Autodesk Fusion 360 part; units mm, degrees
note: some values were not read from the file. Set by a fixed rule: which sketch regions a step uses.
(part 5 of 6)
  line L3690 (386, -69.8094) -> (388, -68.6547)
  line L3691 (362, -93.3453) -> (362, -95.6547)
  line L3692 (391.5, -65.1906) -> (389.5, -66.3453)
  line L3693 (385.25, -90.8916) -> (385.25, -88.5822)
  line L3694 (396.25, -61.5822) -> (394.25, -60.4275)
  line L3695 (391.5, -65.1906) -> (389.5, -66.3453)
  line L3696 (399.75, -65.0463) -> (401.75, -63.8916)
  line L3697 (388.75, -101.0463) -> (390.75, -99.8916)
  line L3698 (388.75, -69.4275) -> (386.75, -70.5822)
  line L3699 (397, -60.8094) -> (399, -59.6547)
  line L3700 (374.25, -61.5822) -> (372.25, -60.4275)
  line L3701 (395, -59.6547) -> (397, -60.8094)
  line L3702 (402.5, -65.1906) -> (400.5, -66.3453)
  line L3703 (404.1665, -57.1527) -> (402.5, -56.1906)
  line L3704 (389.5, -93.3453) -> (389.5, -95.6547)
  line L3705 (386.75, -90.8916) -> (388.75, -92.0463)
  line L3706 (401.75, -63.8916) -> (401.75, -61.5822)
  line L3707 (366, -102.3453) -> (364, -101.1906)
  line L3708 (397.75, -61.5822) -> (397.75, -63.8916)
  line L3709 (373, -59.6547) -> (375, -60.8094)
  line L3710 (388.75, -65.0463) -> (390.75, -63.8916)
  line L3711 (379.75, -90.8916) -> (379.75, -88.5822)
  line L3712 (399.75, -60.4275) -> (397.75, -61.5822)
  line L3713 (386.75, -97.5822) -> (386.75, -99.8916)
  line L3714 (379.75, -54.8916) -> (379.75, -52.5822)
  line L3715 (373, -68.6547) -> (375, -69.8094)
  line L3716 (362, -93.3453) -> (362, -95.6547)
  line L3717 (374.25, -70.5822) -> (372.25, -69.4275)
  line L3718 (374.25, -61.5822) -> (372.25, -60.4275)
  line L3719 (397, -65.1906) -> (395, -66.3453)
  line L3720 (372.25, -65.0463) -> (374.25, -63.8916)
  line L3721 (359.25, -70.5822) -> (359.25, -72.8916)
  line L3722 (386.75, -90.8916) -> (388.75, -92.0463)
  line L3723 (379.75, -90.8916) -> (379.75, -88.5822)
  line L3724 (385.25, -54.8916) -> (385.25, -52.5822)
  line L3725 (401.75, -63.8916) -> (401.75, -61.5822)
  line L3726 (388.75, -65.0463) -> (390.75, -63.8916)
  line L3727 (386.75, -52.5822) -> (386.75, -54.8916)
  line L3728 (375.75, -52.5822) -> (375.75, -54.8916)
  line L3729 (375, -65.1906) -> (373, -66.3453)
  line L3730 (367.5, -93.3453) -> (367.5, -95.6547)
  line L3731 (372.25, -69.4275) -> (370.25, -70.5822)
  line L3732 (375.75, -88.5822) -> (375.75, -90.8916)
  line L3733 (358.5, -87.8094) -> (360.5, -86.6547)
  line L3734 (368.75, -81.8916) -> (368.75, -79.5822)
  line L3735 (364, -96.8094) -> (366, -95.6547)
  line L3736 (373, -66.3453) -> (373, -68.6547)
  line L3737 (388, -66.3453) -> (386, -65.1906)
  line L3738 (377.75, -101.0463) -> (379.75, -99.8916)
  line L3739 (392.25, -70.5822) -> (392.25, -72.8916)
  line L3740 (355.75, -87.4275) -> (353.75, -88.5822)
  line L3741 (379.75, -99.8916) -> (379.75, -97.5822)
  line L3742 (357.75, -72.8916) -> (357.75, -70.5822)
  line L3743 (394.25, -56.0463) -> (396.25, -54.8916)
  line L3744 (362, -84.3453) -> (362, -86.6547)
  line L3745 (402.5, -60.8094) -> (404.5, -59.6547)
  line L3746 (386.75, -70.5822) -> (386.75, -72.8916)
  line L3747 (386, -65.1906) -> (384, -66.3453)
  line L3748 (374.25, -72.8916) -> (374.25, -70.5822)
  line L3749 (366.75, -92.0463) -> (368.75, -90.8916)
  line L3750 (364, -92.1906) -> (362, -93.3453)
  line L3751 (356.5, -86.6547) -> (358.5, -87.8094)
  line L3752 (386.75, -88.5822) -> (386.75, -90.8916)
  line L3753 (370.25, -70.5822) -> (370.25, -72.8916)
  line L3754 (374.25, -72.8916) -> (374.25, -70.5822)
  line L3755 (386.75, -52.5822) -> (386.75, -54.8916)
  line L3756 (390.75, -90.8916) -> (390.75, -88.5822)
  line L3757 (370.25, -70.5822) -> (370.25, -72.8916)
  line L3758 (378.5, -93.3453) -> (378.5, -95.6547)
  line L3759 (366.75, -101.0463) -> (368.75, -99.8916)
  line L3760 (358.5, -83.1906) -> (356.5, -84.3453)
  line L3761 (360.5, -84.3453) -> (358.5, -83.1906)
  line L3762 (397.75, -54.8916) -> (399.75, -56.0463)
  line L3763 (392.25, -88.5822) -> (392.25, -90.8916)
  line L3764 (360.5, -84.3453) -> (358.5, -83.1906)
  line L3765 (394.25, -56.0463) -> (396.25, -54.8916)
  line L3766 (388, -66.3453) -> (386, -65.1906)
  line L3767 (360.5, -86.6547) -> (360.5, -84.3453)
  line L3768 (389.5, -66.3453) -> (389.5, -68.6547)
  line L3769 (368.75, -97.5822) -> (366.75, -96.4275)
  line L3770 (385.25, -54.8916) -> (385.25, -52.5822)
  line L3771 (404.5, -66.3453) -> (402.5, -65.1906)
  line L3772 (379.75, -54.8916) -> (379.75, -52.5822)
  line L3773 (377.75, -92.0463) -> (379.75, -90.8916)
  line L3774 (399.75, -56.0463) -> (401.75, -54.8916)
  line L3775 (355, -86.6547) -> (355, -84.3453)
  line L3776 (401.75, -54.8916) -> (401.75, -53.9293)
  line L3777 (363.25, -81.8916) -> (363.25, -79.5822)
  line L3778 (390.75, -70.5822) -> (388.75, -69.4275)
  line L3779 (401.75, -54.8916) -> (401.75, -53.9293)
  line L3780 (385.25, -72.8916) -> (385.25, -70.5822)
  line L3781 (373, -66.3453) -> (373, -68.6547)
  line L3782 (390.75, -90.8916) -> (390.75, -88.5822)
  line L3783 (372.25, -60.4275) -> (370.25, -61.5822)
  line L3784 (370.25, -61.5822) -> (370.25, -63.8916)
  line L3785 (384, -66.3453) -> (384, -68.6547)
  line L3786 (366.75, -92.0463) -> (368.75, -90.8916)
  line L3787 (364, -92.1906) -> (362, -93.3453)
  line L3788 (360.5, -86.6547) -> (360.5, -84.3453)
  line L3789 (364, -101.1906) -> (362, -102.3453)
  line L3790 (367.5, -93.3453) -> (367.5, -95.6547)
  line L3791 (366.75, -101.0463) -> (368.75, -99.8916)
  line L3792 (370.25, -79.5822) -> (370.25, -81.8916)
  line L3793 (363.25, -99.8916) -> (363.25, -97.5822)
  line L3794 (364.75, -79.5822) -> (364.75, -81.8916)
  line L3795 (386.75, -88.5822) -> (386.75, -90.8916)
  line L3796 (379.75, -97.5822) -> (377.75, -96.4275)
  line L3797 (364.75, -97.5822) -> (364.75, -99.8916)
  line L3798 (392.25, -70.5822) -> (392.25, -72.8916)
  line L3799 (375.75, -88.5822) -> (375.75, -90.8916)
  line L3800 (374.25, -81.8916) -> (374.25, -79.5822)
  line L3801 (390.75, -72.8916) -> (390.75, -70.5822)
  line L3802 (366, -93.3453) -> (364, -92.1906)
  line L3803 (364.75, -90.8916) -> (366.75, -92.0463)
  line L3804 (381.25, -52.5822) -> (381.25, -54.8916)
  line L3805 (375.75, -97.5822) -> (375.75, -99.8916)
  line L3806 (366, -95.6547) -> (366, -93.3453)
  line L3807 (375.75, -97.5822) -> (375.75, -99.8916)
  line L3808 (386.75, -63.8916) -> (388.75, -65.0463)
  line L3809 (377, -95.6547) -> (377, -93.3453)
  line L3810 (359.25, -81.8916) -> (361.25, -83.0463)
  line L3811 (375.75, -90.8916) -> (377.75, -92.0463)
  line L3812 (399, -59.6547) -> (399, -57.3453)
  line L3813 (368.75, -99.8916) -> (368.75, -97.5822)
  line L3814 (377.75, -96.4275) -> (375.75, -97.5822)
  line L3815 (397, -56.1906) -> (395, -57.3453)
  line L3816 (382.5, -93.3453) -> (380.5, -92.1906)
  line L3817 (352.25, -72.8916) -> (352.25, -70.5822)
  line L3818 (359.25, -81.8916) -> (361.25, -83.0463)
  line L3819 (361.25, -87.4275) -> (359.25, -88.5822)
  line L3820 (400.5, -59.6547) -> (402.5, -60.8094)
  line L3821 (399, -57.3453) -> (397, -56.1906)
  line L3822 (397.75, -54.8916) -> (399.75, -56.0463)
  line L3823 (348.25, -70.5822) -> (348.25, -72.8916)
  line L3824 (362, -84.3453) -> (362, -86.6547)
  line L3825 (397, -56.1906) -> (395, -57.3453)
  line L3826 (399, -57.3453) -> (397, -56.1906)
  line L3827 (378.5, -95.6547) -> (380.5, -96.8094)
  line L3828 (378.5, -95.6547) -> (380.5, -96.8094)
  line L3829 (366.75, -96.4275) -> (364.75, -97.5822)
  line L3830 (388, -68.6547) -> (388, -66.3453)
  line L3831 (389.5, -68.6547) -> (391.5, -69.8094)
  line L3832 (364.75, -97.5822) -> (364.75, -99.8916)
  line L3833 (377.75, -92.0463) -> (379.75, -90.8916)
  line L3834 (381.25, -90.8916) -> (383.25, -92.0463)
  line L3835 (386.75, -63.8916) -> (388.75, -65.0463)
  line L3836 (355, -86.6547) -> (355, -84.3453)
  line L3837 (381.25, -88.5822) -> (381.25, -90.8916)
  line L3838 (366.75, -96.4275) -> (364.75, -97.5822)
  line L3839 (399.75, -56.0463) -> (401.75, -54.8916)
  line L3840 (363.25, -81.8916) -> (363.25, -79.5822)
  line L3841 (390.75, -72.8916) -> (390.75, -70.5822)
  line L3842 (377, -95.6547) -> (377, -93.3453)
  line L3843 (369.5, -60.8094) -> (371.5, -59.6547)
  line L3844 (361.25, -87.4275) -> (359.25, -88.5822)
  line L3845 (388, -68.6547) -> (388, -66.3453)
  line L3846 (362, -95.6547) -> (364, -96.8094)
  line L3847 (368.75, -99.8916) -> (368.75, -97.5822)
  line L3848 (385.25, -72.8916) -> (385.25, -70.5822)
  line L3849 (364.75, -79.5822) -> (364.75, -81.8916)
  line L3850 (389.5, -68.6547) -> (391.5, -69.8094)
  line L3851 (371.5, -66.3453) -> (369.5, -65.1906)
  line L3852 (356.5, -86.6547) -> (358.5, -87.8094)
  line L3853 (366, -102.3453) -> (364, -101.1906)
  line L3854 (364.75, -90.8916) -> (366.75, -92.0463)
  line L3855 (364, -96.8094) -> (366, -95.6547)
  line L3856 (399, -59.6547) -> (399, -57.3453)
  line L3857 (353.75, -81.8916) -> (355.75, -83.0463)
  line L3858 (358.5, -83.1906) -> (356.5, -84.3453)
  line L3859 (366, -93.3453) -> (364, -92.1906)
  line L3860 (393.5, -59.6547) -> (393.5, -57.3453)
  line L3861 (358.5, -87.8094) -> (360.5, -86.6547)
  line L3862 (384, -68.6547) -> (386, -69.8094)
  line L3863 (364.75, -99.8916) -> (366.75, -101.0463)
  line L3864 (371.5, -57.3453) -> (369.5, -56.1906)
  line L3865 (381.25, -52.5822) -> (381.25, -54.8916)
  line L3866 (357.75, -88.5822) -> (355.75, -87.4275)
  line L3867 (373, -41.6547) -> (375, -42.8094)
  line L3868 (381.25, -97.5822) -> (381.25, -99.8916)
  line L3869 (364, -101.1906) -> (362, -102.3453)
  line L3870 (372.25, -42.4275) -> (370.25, -43.5822)
  line L3871 (355.75, -83.0463) -> (357.75, -81.8916)
  line L3872 (372.25, -51.4275) -> (370.25, -52.5822)
  line L3873 (380.5, -92.1906) -> (378.5, -93.3453)
  line L3874 (393.5, -59.6547) -> (393.5, -57.3453)
  line L3875 (369.5, -51.8094) -> (371.5, -50.6547)
  line L3876 (392.25, -52.5822) -> (392.25, -54.8916)
  line L3877 (372.25, -42.4275) -> (370.25, -43.5822)
  line L3878 (357.75, -72.8916) -> (357.75, -70.5822)
  line L3879 (386.75, -70.5822) -> (386.75, -72.8916)
  line L3880 (388.75, -69.4275) -> (386.75, -70.5822)
  line L3881 (366, -95.6547) -> (366, -93.3453)
  line L3882 (355.75, -83.0463) -> (357.75, -81.8916)
  line L3883 (375.75, -90.8916) -> (377.75, -92.0463)
  line L3884 (368.75, -97.5822) -> (366.75, -96.4275)
  line L3885 (386, -65.1906) -> (384, -66.3453)
  line L3886 (384, -66.3453) -> (384, -68.6547)
  line L3887 (383.25, -78.4275) -> (381.25, -79.5822)
  line L3888 (390.75, -70.5822) -> (388.75, -69.4275)
  line L3889 (375, -56.1906) -> (373, -57.3453)
  line L3890 (381.25, -99.8916) -> (383.25, -101.0463)
  line L3891 (357.75, -88.5822) -> (355.75, -87.4275)
  line L3892 (402.5, -56.1906) -> (400.5, -57.3453)
  line L3893 (374.25, -45.8916) -> (374.25, -43.5822)
  line L3894 (371.5, -57.3453) -> (369.5, -56.1906)
  line L3895 (356.5, -84.3453) -> (356.5, -86.6547)
  line L3896 (380.5, -96.8094) -> (382.5, -95.6547)
  line L3897 (379.75, -99.8916) -> (379.75, -97.5822)
  line L3898 (370.25, -52.5822) -> (370.25, -54.8916)
  line L3899 (404.5, -66.3453) -> (402.5, -65.1906)
  line L3900 (400.5, -57.3453) -> (400.5, -59.6547)
  line L3901 (402.5, -56.1906) -> (400.5, -57.3453)
  line L3902 (371.5, -50.6547) -> (371.5, -48.3453)
  line L3903 (356.5, -84.3453) -> (356.5, -86.6547)
  line L3904 (382.5, -95.6547) -> (382.5, -93.3453)
  line L3905 (362, -95.6547) -> (364, -96.8094)
  line L3906 (381.25, -97.5822) -> (381.25, -99.8916)
  line L3907 (386, -69.8094) -> (388, -68.6547)
  line L3908 (395, -57.3453) -> (395, -59.6547)
  line L3909 (382.5, -93.3453) -> (380.5, -92.1906)
  line L3910 (355.75, -87.4275) -> (353.75, -88.5822)
  line L3911 (377.75, -101.0463) -> (379.75, -99.8916)
  line L3912 (353.75, -70.5822) -> (353.75, -72.8916)
  line L3913 (364.75, -99.8916) -> (366.75, -101.0463)
  line L3914 (389.5, -66.3453) -> (389.5, -68.6547)
  line L3915 (400.5, -59.6547) -> (402.5, -60.8094)
  line L3916 (400.5, -57.3453) -> (400.5, -59.6547)
  line L3917 (374.25, -52.5822) -> (372.25, -51.4275)
  line L3918 (381.25, -81.8916) -> (383.25, -83.0463)
  line L3919 (370.25, -43.5822) -> (370.25, -45.8916)
  line L3920 (369.5, -60.8094) -> (371.5, -59.6547)
  line L3921 (395, -57.3453) -> (395, -59.6547)
  line L3922 (375.75, -99.8916) -> (377.75, -101.0463)
  line L3923 (383.25, -87.4275) -> (381.25, -88.5822)
  line L3924 (352.25, -72.8916) -> (352.25, -70.5822)
  line L3925 (346.75, -72.8916) -> (346.75, -70.5822)
  line L3926 (375.75, -52.5822) -> (375.75, -54.8916)
  line L3927 (346.75, -72.8916) -> (346.75, -70.5822)
  line L3928 (370.25, -43.5822) -> (370.25, -45.8916)
  line L3929 (356.5, -77.6547) -> (358.5, -78.8094)
  line L3930 (378.5, -93.3453) -> (378.5, -95.6547)
  line L3931 (385.25, -88.5822) -> (383.25, -87.4275)
  line L3932 (370.25, -45.8916) -> (372.25, -47.0463)
  line L3933 (372.25, -47.0463) -> (374.25, -45.8916)
  line L3934 (369.5, -42.8094) -> (371.4564, -41.6798)
  line L3935 (388.75, -87.4275) -> (386.75, -88.5822)
  line L3936 (379.75, -97.5822) -> (377.75, -96.4275)
  line L3937 (390.75, -88.5822) -> (388.75, -87.4275)
  line L3938 (375, -56.1906) -> (373, -57.3453)
  line L3939 (353, -78.8094) -> (355, -77.6547)
  line L3940 (348.25, -70.5822) -> (348.25, -72.8916)
  line L3941 (386, -83.1906) -> (384, -84.3453)
  line L3942 (372.25, -56.0463) -> (374.25, -54.8916)
  line L3943 (355, -75.3453) -> (353, -74.1906)
  line L3944 (371.5, -75.3453) -> (369.5, -74.1906)
  line L3945 (384, -84.3453) -> (384, -86.6547)
  line L3946 (369.5, -42.8094) -> (371.4564, -41.6798)
  line L3947 (385.25, -97.5822) -> (383.25, -96.4275)
  line L3948 (361.25, -78.4275) -> (359.25, -79.5822)
  line L3949 (381.25, -90.8916) -> (383.25, -92.0463)
  line L3950 (375, -47.1906) -> (373, -48.3453)
  line L3951 (372.25, -56.0463) -> (374.25, -54.8916)
  line L3952 (374.25, -54.8916) -> (374.25, -52.5822)
  line L3953 (355.75, -78.4275) -> (353.75, -79.5822)
  line L3954 (383.25, -92.0463) -> (385.25, -90.8916)
  line L3955 (385.25, -79.5822) -> (383.25, -78.4275)
  line L3956 (381.25, -99.8916) -> (383.25, -101.0463)
  line L3957 (380.5, -92.1906) -> (378.5, -93.3453)
  line L3958 (382.5, -68.6547) -> (382.5, -66.3453)
  line L3959 (352.25, -54.8916) -> (352.25, -52.5822)
  line L3960 (357.75, -79.5822) -> (355.75, -78.4275)
  line L3961 (389.5, -84.3453) -> (389.5, -86.6547)
  line L3962 (370.25, -45.8916) -> (372.25, -47.0463)
  line L3963 (373, -41.5572) -> (373, -41.6547)
  line L3964 (385.25, -79.5822) -> (383.25, -78.4275)
  line L3965 (375.75, -99.8916) -> (377.75, -101.0463)
  line L3966 (383.25, -83.0463) -> (385.25, -81.8916)
  line L3967 (386.75, -81.8916) -> (388.75, -83.0463)
  line L3968 (383.25, -87.4275) -> (381.25, -88.5822)
  line L3969 (388, -86.6547) -> (388, -84.3453)
  line L3970 (382.5, -95.6547) -> (382.5, -93.3453)
  line L3971 (375.75, -70.5822) -> (375.75, -72.8916)
  line L3972 (383.25, -96.4275) -> (381.25, -97.5822)
  line L3973 (383.25, -96.4275) -> (381.25, -97.5822)
  line L3974 (377.75, -65.0463) -> (379.75, -63.8916)
  line L3975 (381.25, -70.5822) -> (381.25, -72.8916)
  line L3976 (383.25, -101.0463) -> (385.25, -99.8916)
  line L3977 (377.75, -96.4275) -> (375.75, -97.5822)
  line L3978 (381.25, -81.8916) -> (383.25, -83.0463)
  line L3979 (355, -77.6547) -> (355, -75.3453)
  line L3980 (383.25, -83.0463) -> (385.25, -81.8916)
  line L3981 (359.25, -70.5822) -> (359.25, -72.8916)
  line L3982 (388, -86.6547) -> (388, -84.3453)
  line L3983 (353, -78.8094) -> (355, -77.6547)
  line L3984 (360.5, -75.3453) -> (358.5, -74.1906)
  line L3985 (390.75, -88.5822) -> (388.75, -87.4275)
  arc A135 (371.4564, -41.6798) -> (368.3398, -42.1395) centre (375, -76.5) ccw
  line L3986 (388, -84.3453) -> (386, -83.1906)
  line L3987 (369.5, -69.8094) -> (371.5, -68.6547)
  line L3988 (373, -48.3453) -> (373, -50.6547)
  line L3989 (380.5, -96.8094) -> (382.5, -95.6547)
  line L3990 (382.5, -68.6547) -> (382.5, -66.3453)
  line L3991 (389.5, -84.3453) -> (389.5, -86.6547)
  line L3992 (373, -50.6547) -> (375, -51.8094)
  line L3993 (383.25, -101.0463) -> (385.25, -99.8916)
  line L3994 (358.5, -74.1906) -> (356.5, -75.3453)
  line L3995 (360.5, -77.6547) -> (360.5, -75.3453)
  line L3996 (358.5, -78.8094) -> (360.5, -77.6547)
  line L3997 (370.25, -54.8916) -> (372.25, -56.0463)
  line L3998 (375.75, -70.5822) -> (375.75, -72.8916)
  line L3999 (371.5, -50.6547) -> (371.5, -48.3453)
  line L4000 (389.5, -86.6547) -> (391.5, -87.8094)
  line L4001 (375.75, -63.8916) -> (377.75, -65.0463)
  line L4002 (388.75, -83.0463) -> (390.75, -81.8916)
  line L4003 (386, -87.8094) -> (388, -86.6547)
  line L4004 (379.75, -72.8916) -> (379.75, -70.5822)
  line L4005 (378.5, -66.3453) -> (378.5, -68.6547)
  line L4006 (374.25, -45.8916) -> (374.25, -43.5822)
  line L4007 (386.75, -61.5822) -> (386.75, -63.8916)
  line L4008 (389.5, -86.6547) -> (391.5, -87.8094)
  line L4009 (370.25, -54.8916) -> (372.25, -56.0463)
  line L4010 (362, -75.3453) -> (362, -77.6547)
  line L4011 (384, -84.3453) -> (384, -86.6547)
  line L4012 (360.5, -75.3453) -> (358.5, -74.1906)
  line L4013 (379.75, -45.8916) -> (379.75, -43.5822)
  line L4014 (369.5, -78.8094) -> (371.5, -77.6547)
  line L4015 (358.5, -74.1906) -> (356.5, -75.3453)
  line L4016 (377, -68.6547) -> (377, -66.3453)
  line L4017 (388.75, -87.4275) -> (386.75, -88.5822)
  line L4018 (360.5, -68.6547) -> (360.5, -66.3453)
  line L4019 (391.5, -83.1906) -> (389.5, -84.3453)
  line L4020 (383.25, -78.4275) -> (381.25, -79.5822)
  line L4021 (372.25, -47.0463) -> (374.25, -45.8916)
  line L4022 (371.5, -66.3453) -> (369.5, -65.1906)
  line L4023 (355, -84.3453) -> (353, -83.1906)
  line L4024 (359.25, -52.5822) -> (359.25, -54.8916)
  line L4025 (391.5, -83.1906) -> (389.5, -84.3453)
  line L4026 (374.25, -43.5822) -> (372.25, -42.4275)
  line L4027 (377.75, -69.4275) -> (375.75, -70.5822)
  line L4028 (386, -87.8094) -> (388, -86.6547)
  line L4029 (348.25, -53.9293) -> (348.25, -54.8916)
  line L4030 (374.25, -54.8916) -> (374.25, -52.5822)
  line L4031 (381.25, -70.5822) -> (381.25, -72.8916)
  line L4032 (385.25, -88.5822) -> (383.25, -87.4275)
  line L4033 (373, -41.5572) -> (373, -41.6547)
  line L4034 (380.5, -69.8094) -> (382.5, -68.6547)
  line L4035 (355.75, -65.0463) -> (357.75, -63.8916)
  line L4036 (382.5, -66.3453) -> (380.5, -65.1906)
  line L4037 (355.75, -78.4275) -> (353.75, -79.5822)
  line L4038 (369.5, -51.8094) -> (371.5, -50.6547)
  line L4039 (371.5, -75.3453) -> (369.5, -74.1906)
  line L4040 (369.5, -78.8094) -> (371.5, -77.6547)
  line L4041 (353.75, -72.8916) -> (355.75, -74.0463)
  line L4042 (373, -50.6547) -> (375, -51.8094)
  line L4043 (379.75, -72.8916) -> (379.75, -70.5822)
  line L4044 (357.75, -54.8916) -> (357.75, -52.5822)
  line L4045 (358.5, -78.8094) -> (360.5, -77.6547)
  line L4046 (383.25, -92.0463) -> (385.25, -90.8916)
  line L4047 (390.75, -81.8916) -> (390.75, -79.5822)
  line L4048 (385.25, -97.5822) -> (383.25, -96.4275)
  line L4049 (373, -48.3453) -> (373, -50.6547)
  line L4050 (356.5, -66.3453) -> (356.5, -68.6547)
  line L4051 (353, -87.8094) -> (355, -86.6547)
  line L4052 (355, -77.6547) -> (355, -75.3453)
  line L4053 (384, -86.6547) -> (386, -87.8094)
  line L4054 (377, -68.6547) -> (377, -66.3453)
  line L4055 (382.5, -84.3453) -> (380.5, -83.1906)
  line L4056 (388, -84.3453) -> (386, -83.1906)
  line L4057 (373, -57.3453) -> (373, -59.6547)
  line L4058 (388, -48.3453) -> (386, -47.1906)
  line L4059 (360.5, -77.6547) -> (360.5, -75.3453)
  line L4060 (372.25, -51.4275) -> (370.25, -52.5822)
  line L4061 (379.75, -63.8916) -> (379.75, -61.5822)
  line L4062 (359.25, -72.8916) -> (361.25, -74.0463)
  line L4063 (357.75, -70.5822) -> (355.75, -69.4275)
  line L4064 (392.25, -79.5822) -> (392.25, -81.8916)
  line L4065 (375, -47.1906) -> (373, -48.3453)
  line L4066 (356.5, -68.6547) -> (358.5, -69.8094)
  line L4067 (362, -66.3453) -> (362, -68.6547)
  line L4068 (373, -41.6547) -> (375, -42.8094)
  line L4069 (362, -66.3453) -> (362, -68.6547)
  line L4070 (355.75, -74.0463) -> (357.75, -72.8916)
  line L4071 (375.75, -63.8916) -> (377.75, -65.0463)
  line L4072 (378.5, -86.6547) -> (380.5, -87.8094)
  line L4073 (356.5, -68.6547) -> (358.5, -69.8094)
  line L4074 (382.5, -84.3453) -> (380.5, -83.1906)
  line L4075 (386, -83.1906) -> (384, -84.3453)
  line L4076 (359.25, -63.8916) -> (361.25, -65.0463)
  line L4077 (392.25, -79.5822) -> (392.25, -81.8916)
  line L4078 (384, -86.6547) -> (386, -87.8094)
  line L4079 (386.75, -45.8916) -> (388.75, -47.0463)
  line L4080 (378.5, -68.6547) -> (380.5, -69.8094)
  line L4081 (359.25, -63.8916) -> (361.25, -65.0463)
  line L4082 (385.25, -81.8916) -> (385.25, -79.5822)
  line L4083 (386, -47.1906) -> (384, -48.3453)
  line L4084 (377, -86.6547) -> (377, -84.3453)
  line L4085 (371.5, -59.6547) -> (371.5, -57.3453)
  line L4086 (380.5, -69.8094) -> (382.5, -68.6547)
  line L4087 (379.75, -70.5822) -> (377.75, -69.4275)
  line L4088 (374.25, -43.5822) -> (372.25, -42.4275)
  line L4089 (381.25, -43.5822) -> (381.25, -45.8916)
  line L4090 (357.75, -79.5822) -> (355.75, -78.4275)
  line L4091 (379.75, -63.8916) -> (379.75, -61.5822)
  line L4092 (359.25, -72.8916) -> (361.25, -74.0463)
  line L4093 (386.75, -81.8916) -> (388.75, -83.0463)
  line L4094 (361.25, -69.4275) -> (359.25, -70.5822)
  line L4095 (389.5, -50.6547) -> (391.5, -51.8094)
  line L4096 (380.5, -65.1906) -> (378.5, -66.3453)
  line L4097 (357.75, -70.5822) -> (355.75, -69.4275)
  line L4098 (390.75, -81.8916) -> (390.75, -79.5822)
  line L4099 (361.25, -78.4275) -> (359.25, -79.5822)
  line L4100 (375.75, -43.5822) -> (375.75, -45.8916)
  line L4101 (374.25, -52.5822) -> (372.25, -51.4275)
  line L4102 (375.75, -81.8916) -> (377.75, -83.0463)
  line L4103 (370.25, -52.5822) -> (370.25, -54.8916)
  line L4104 (382.5, -66.3453) -> (380.5, -65.1906)
  line L4105 (381.25, -43.5822) -> (381.25, -45.8916)
  line L4106 (377.75, -65.0463) -> (379.75, -63.8916)
  line L4107 (388.75, -83.0463) -> (390.75, -81.8916)
  line L4108 (356.5, -75.3453) -> (356.5, -77.6547)
  line L4109 (362, -75.3453) -> (362, -77.6547)
  line L4110 (373, -57.3453) -> (373, -59.6547)
  line L4111 (377.75, -87.4275) -> (375.75, -88.5822)
  line L4112 (379.75, -70.5822) -> (377.75, -69.4275)
  line L4113 (378.5, -68.6547) -> (380.5, -69.8094)
  line L4114 (356.5, -75.3453) -> (356.5, -77.6547)
  line L4115 (361.25, -69.4275) -> (359.25, -70.5822)
  arc A136 (371.4564, -41.6798) -> (368.3398, -42.1395) centre (375, -76.5) ccw
  line L4116 (379.75, -88.5822) -> (377.75, -87.4275)
  line L4117 (380.5, -65.1906) -> (378.5, -66.3453)
  line L4118 (355.75, -74.0463) -> (357.75, -72.8916)
  line L4119 (360.5, -66.3453) -> (358.5, -65.1906)
  line L4120 (377.75, -69.4275) -> (375.75, -70.5822)
  line L4121 (382.5, -86.6547) -> (382.5, -84.3453)
  line L4122 (353.75, -52.5822) -> (353.75, -54.8916)
  line L4123 (356.5, -77.6547) -> (358.5, -78.8094)
  line L4124 (388.75, -51.4275) -> (386.75, -52.5822)
  line L4125 (389.5, -48.3453) -> (389.5, -50.6547)
  line L4126 (371.5, -59.6547) -> (371.5, -57.3453)
  line L4127 (353.75, -63.8916) -> (355.75, -65.0463)
  arc A137 (387.3612, -109.2445) -> (390.75, -107.756) centre (375, -76.5) ccw
  arc A138 (387.3612, -109.2445) -> (390.75, -107.756) centre (375, -76.5) ccw
  line L4128 (388.75, -105.4275) -> (386.75, -106.5822)
  line L4129 (390.75, -106.5822) -> (388.75, -105.4275)
  line L4130 (384, -104.6547) -> (386, -105.8094)
  line L4131 (388, -104.6547) -> (388, -102.3453)
  line L4132 (380.5, -105.8094) -> (382.5, -104.6547)
  line L4133 (381.25, -106.5822) -> (381.25, -108.8916)
  line L4134 (386.75, -106.5822) -> (386.75, -108.8916)
  line L4135 (380.5, -105.8094) -> (382.5, -104.6547)
  line L4136 (375.75, -106.5822) -> (375.75, -108.8916)
  line L4137 (386, -105.8094) -> (388, -104.6547)
  line L4138 (379.75, -106.5822) -> (377.75, -105.4275)
  line L4139 (379.75, -108.8916) -> (379.75, -106.5822)
  line L4140 (386.75, -106.5822) -> (386.75, -108.8916)
  line L4141 (375.75, -106.5822) -> (375.75, -108.8916)
  line L4142 (381.25, -106.5822) -> (381.25, -108.8916)
  line L4143 (388.75, -105.4275) -> (386.75, -106.5822)
  line L4144 (379.75, -108.8916) -> (379.75, -106.5822)
  line L4145 (385.25, -108.8916) -> (385.25, -106.5822)
  line L4146 (375, -60.8094) -> (377, -59.6547)
  line L4147 (390.75, -106.5822) -> (388.75, -105.4275)
  line L4148 (385.25, -108.8916) -> (385.25, -106.5822)
  line L4149 (402.5, -96.8094) -> (404.1665, -95.8473)
  line L4150 (400.5, -95.6547) -> (402.5, -96.8094)
  line L4151 (404.5, -93.3453) -> (402.5, -92.1906)
  line L4152 (402.5, -87.8094) -> (404.5, -86.6547)
  line L4153 (400.5, -95.6547) -> (402.5, -96.8094)
  line L4154 (402.5, -92.1906) -> (400.5, -93.3453)
  line L4155 (404.5, -93.3453) -> (402.5, -92.1906)
  line L4156 (400.5, -86.6547) -> (402.5, -87.8094)
  line L4157 (395, -93.3453) -> (395, -95.6547)
  line L4158 (399, -95.6547) -> (399, -93.3453)
  line L4159 (395, -93.3453) -> (395, -95.6547)
  line L4160 (393.5, -95.6547) -> (393.5, -93.3453)
  line L4161 (400.5, -93.3453) -> (400.5, -95.6547)
  line L4162 (402.5, -92.1906) -> (400.5, -93.3453)
  line L4163 (393.5, -95.6547) -> (393.5, -93.3453)
  line L4164 (402.5, -87.8094) -> (404.5, -86.6547)
  line L4165 (400.5, -93.3453) -> (400.5, -95.6547)
  line L4166 (391.5, -105.8094) -> (393.5, -104.6547)
  line L4167 (389.5, -104.6547) -> (391.5, -105.8094)
  line L4168 (393.5, -104.6547) -> (393.5, -102.3453)
  line L4169 (390.75, -107.756) -> (390.75, -106.5822)
  line L4170 (393.5, -104.6547) -> (393.5, -102.3453)
  line L4171 (392.25, -106.5822) -> (392.25, -106.9539)
  line L4172 (391.5, -105.8094) -> (393.5, -104.6547)
  line L4173 (390.75, -107.756) -> (390.75, -106.5822)
  line L4174 (389.5, -104.6547) -> (391.5, -105.8094)
  line L4175 (389.5, -102.3453) -> (389.5, -104.6547)
  line L4176 (392.25, -106.5822) -> (392.25, -106.9539)
  line L4177 (399.75, -87.4275) -> (397.75, -88.5822)
  line L4178 (399.75, -92.0463) -> (401.75, -90.8916)
  line L4179 (397, -92.1906) -> (395, -93.3453)
  line L4180 (395, -86.6547) -> (397, -87.8094)
  line L4181 (394.25, -92.0463) -> (396.25, -90.8916)
  line L4182 (395, -86.6547) -> (397, -87.8094)
  line L4183 (397.75, -88.5822) -> (397.75, -90.8916)
  line L4184 (401.75, -90.8916) -> (401.75, -88.5822)
  line L4185 (396.25, -90.8916) -> (396.25, -88.5822)
  line L4186 (397, -87.8094) -> (399, -86.6547)
  line L4187 (401.75, -88.5822) -> (399.75, -87.4275)
  line L4188 (397, -87.8094) -> (399, -86.6547)
  line L4189 (397.75, -88.5822) -> (397.75, -90.8916)
  line L4190 (397.75, -90.8916) -> (399.75, -92.0463)
  line L4191 (397, -92.1906) -> (395, -93.3453)
  line L4192 (399, -95.6547) -> (399, -93.3453)
  line L4193 (399, -93.3453) -> (397, -92.1906)
  line L4194 (399.75, -87.4275) -> (397.75, -88.5822)
  line L4195 (399.75, -92.0463) -> (401.75, -90.8916)
  line L4196 (396.25, -88.5822) -> (394.25, -87.4275)
  line L4197 (394.25, -92.0463) -> (396.25, -90.8916)
  line L4198 (405.25, -87.4275) -> (403.25, -88.5822)
  line L4199 (405.25, -87.4275) -> (403.25, -88.5822)
  line L4200 (403.25, -90.8916) -> (405.25, -92.0463)
  arc A139 (377, -41.5572) -> (373, -41.5572) centre (375, -76.5) ccw
  line L4201 (403.25, -88.5822) -> (403.25, -90.8916)
  line L4202 (407.25, -88.5822) -> (405.25, -87.4275)
  arc A140 (406.7807, -91.1625) -> (407.25, -90.0992) centre (375, -76.5) ccw
  arc A141 (406.7807, -91.1625) -> (407.25, -90.0992) centre (375, -76.5) ccw
  line L4203 (405.25, -92.0463) -> (406.7807, -91.1625)
  line L4204 (408, -87.8094) -> (408.1524, -87.7214)
  line L4205 (407.25, -90.0992) -> (407.25, -88.5822)
  arc A142 (404.1665, -95.8473) -> (404.5, -95.3348) centre (375, -76.5) ccw
  line L4206 (403.25, -88.5822) -> (403.25, -90.8916)
  line L4207 (406, -86.6547) -> (408, -87.8094)
  line L4208 (403.25, -90.8916) -> (405.25, -92.0463)
  arc A143 (404.1665, -95.8473) -> (404.5, -95.3348) centre (375, -76.5) ccw
  line L4209 (405.25, -92.0463) -> (406.7807, -91.1625)
  line L4210 (407.25, -88.5822) -> (405.25, -87.4275)
  line L4211 (408, -87.8094) -> (408.1524, -87.7214)
  line L4212 (404.5, -95.3348) -> (404.5, -93.3453)
  line L4213 (406, -86.6547) -> (408, -87.8094)
  line L4214 (404.5, -95.3348) -> (404.5, -93.3453)
  line L4215 (407.25, -90.0992) -> (407.25, -88.5822)
  line L4216 (547.7721, 225.15) -> (517.5279, 225.15)
  arc A144 (553.8, 219.1221) -> (547.7721, 225.15) centre (532.65, 204) ccw
  line L4217 (553.8, 219.1221) -> (553.8, 188.8779)
  arc A145 (547.7721, 182.85) -> (553.8, 188.8779) centre (532.65, 204) ccw
  line L4218 (547.7721, 182.85) -> (517.5279, 182.85)
  arc A146 (511.5, 188.8779) -> (517.5279, 182.85) centre (532.65, 204) ccw
  line L4219 (511.5, 188.8779) -> (511.5, 219.1221)
  circle A147 centre (517.15, 188.5) radius 1.5
  circle A148 centre (548.15, 188.5) radius 1.5
  circle A149 centre (517.15, 219.5) radius 1.5
  circle A150 centre (548.15, 219.5) radius 1.5
  arc A151 (517.5279, 225.15) -> (511.5, 219.1221) centre (532.65, 204) ccw
  circle A152 centre (405.0052, 247.5049) radius 2
  circle A153 centre (345.0052, 247.5049) radius 2
  circle A154 centre (345.0052, 187.5049) radius 2
  circle A155 centre (405.0052, 187.5049) radius 2
  circle A156 centre (345.0026, -46.496) radius 2
  circle A157 centre (405.0026, -46.496) radius 2
  circle A158 centre (345.0026, -106.496) radius 2
  circle A159 centre (405.0026, -106.496) radius 2
  line L4220 (641.1, -21.5) -> (730.1, -21.5)
  line L4221 (730.1, -21.5) -> (730.1, -63.5)
  line L4222 (730.1, -63.5) -> (641.1, -63.5)
  line L4223 (641.1, -63.5) -> (641.1, -21.5)
  line L4224 (635.6, -119.5) -> (645.6, -119.5)
  line L4225 (645.6, -119.5) -> (645.6, -94)
  line L4226 (645.6, -94) -> (635.6, -94)
  line L4227 (635.6, -94) -> (635.6, -119.5)
  line L4228 (723.6, -94) -> (733.6, -94)
  line L4229 (733.6, -94) -> (733.6, -119.5)
  line L4230 (733.6, -119.5) -> (723.6, -119.5)
  line L4231 (723.6, -119.5) -> (723.6, -94)
  circle A160 centre (684.6183, -98.5274) radius 17.5
  line L4232 (620, -10) -> (749.2, -10)
  line L4233 (699.45, -122) -> (699.45, -125)
  line L4234 (721.95, -122) -> (744.4305, -122)
  line L4235 (749.2, -122) -> (749.2, -10)
  line L4236 (676.95, -122) -> (699.45, -122)
  line L4237 (721.95, -125) -> (721.95, -122)
  line L4238 (620, -125) -> (631.95, -125)
  line L4239 (631.95, -125) -> (631.95, -122)
  line L4240 (631.95, -122) -> (654.45, -122)
  line L4241 (744.4305, -122) -> (749.2, -122)
  line L4242 (620, -10) -> (620, -125)
  line L4243 (676.95, -125) -> (676.95, -122)
  line L4244 (654.45, -122) -> (654.45, -125)
  line L4245 (654.45, -125) -> (676.95, -125)
  line L4246 (699.45, -125) -> (721.95, -125)
  line L4247 (1049.3657, 371.7532) -> (1039.3657, 371.7532)
  line L4248 (1018.1339, 373.7259) -> (982.6339, 373.7259)
  line L4249 (951.3657, 371.7532) -> (961.3657, 371.7532)
  line L4250 (1049.3657, 397.2532) -> (1049.3657, 371.7532)
  line L4251 (1064.4656, 369.2532) -> (936.2656, 369.2532)
  line L4252 (951.3656, 478.7533) -> (951.3656, 418.7533)
  line L4253 (1032.3657, 371.7532) -> (1032.3657, 413.7532)
  line L4254 (968.3657, 371.7532) -> (944.3657, 371.7532)
  circle A161 centre (1000.3839, 392.7259) radius 17
  line L4255 (1056.3657, 371.7532) -> (1032.3657, 371.7532)
  line L4256 (1064.4656, 481.2532) -> (1064.4656, 369.2532)
  line L4257 (982.6339, 411.7259) -> (1018.1339, 411.7259)
  line L4258 (1049.3656, 418.7533) -> (1049.3656, 478.7533)
  line L4259 (1039.3657, 397.2532) -> (1049.3657, 397.2532)
  line L4260 (1049.3656, 478.7533) -> (951.3656, 478.7533)
  line L4261 (936.2656, 481.2532) -> (1064.4656, 481.2532)
  line L4262 (1000.3839, 411.7259) -> (1000.3839, 373.7259)
  line L4263 (944.3657, 392.7532) -> (968.3657, 392.7532)
  line L4264 (968.3657, 413.7532) -> (968.3657, 371.7532)
  line L4265 (982.6339, 373.7259) -> (982.6339, 411.7259)
  line L4266 (944.3657, 413.7532) -> (968.3657, 413.7532)
  line L4267 (961.3657, 397.2532) -> (951.3657, 397.2532)
  line L4268 (1044.3657, 413.7532) -> (1044.3657, 371.7532)
  line L4269 (956.3657, 413.7532) -> (956.3657, 371.7532)
  line L4270 (1000.3656, 478.7533) -> (1000.3656, 418.7533)
  line L4271 (951.3656, 418.7533) -> (1049.3656, 418.7533)
  line L4272 (951.3656, 448.7533) -> (1049.3656, 448.7533)
  line L4273 (1032.3657, 413.7532) -> (1056.3657, 413.7532)
  line L4274 (936.2656, 369.2532) -> (936.2656, 481.2532)
  line L4275 (944.3657, 371.7532) -> (944.3657, 413.7532)
  line L4276 (1018.1339, 411.7259) -> (1018.1339, 373.7259)
  line L4277 (1039.3657, 371.7532) -> (1039.3657, 397.2532)
  line L4278 (1032.3657, 392.7532) -> (1056.3657, 392.7532)
  line L4279 (961.3657, 371.7532) -> (961.3657, 397.2532)
  line L4280 (1056.3657, 413.7532) -> (1056.3657, 371.7532)
  line L4281 (951.3657, 397.2532) -> (951.3657, 371.7532)
  line L4282 (982.6339, 392.7259) -> (1018.1339, 392.7259)
  circle A162 centre (638.12, -15.02) radius 1.25
  circle A163 centre (731.08, -15.02) radius 1.25
  circle A164 centre (731.08, -69.98) radius 1.25
  circle A165 centre (638.12, -69.98) radius 1.25
  circle A166 centre (669.4183, -84.5774) radius 1.25
  circle A167 centre (699.8183, -84.5774) radius 1.25
  circle A168 centre (669.4183, -114.9774) radius 1.25
  circle A169 centre (699.8183, -114.9774) radius 1.25
  line L4283 (450, -10) -> (450, -76)
  line L4284 (578.2, -76) -> (578.2, -64.75)
  line L4285 (506.95, -13) -> (506.95, -10)
  line L4286 (551.95, -13) -> (551.95, -10)
  line L4287 (529.45, -10) -> (529.45, -13)
  line L4288 (484.45, -10) -> (484.45, -13)
  line L4289 (461.95, -10) -> (450, -10)
  line L4290 (484.45, -13) -> (461.95, -13)
  line L4291 (506.95, -10) -> (484.45, -10)
  line L4292 (529.45, -13) -> (506.95, -13)
  line L4293 (578.2, -19.75) -> (578.2, -13)
  line L4294 (551.95, -10) -> (529.45, -10)
  line L4295 (578.2, -13) -> (551.95, -13)
  line L4296 (461.95, -13) -> (461.95, -10)
  line L4297 (450, -76) -> (578.2, -76)
  circle A170 centre (459.2, -22) radius 1.5
  circle A171 centre (459.2, -62) radius 1.5
  circle A172 centre (569.2, -22) radius 1.5
  circle A173 centre (569.2, -62) radius 1.5
  line L4298 (617.8, 135) -> (608.25, 135)
  line L4299 (608.25, 3) -> (617.8, 3)
  line L4300 (173.8, 285) -> (173.8, 381.147)
  line L4301 (173.8, 381.147) -> (186.75, 381.147)
  line L4302 (375, 90.147) -> (386.25, 90.147)
  line L4303 (578.2, -64.75) -> (581.2, -64.75)
  line L4304 (581.2, -64.75) -> (581.2, -42.25)
  line L4305 (581.2, -42.25) -> (578.2, -42.25)
  line L4306 (578.2, -42.25) -> (578.2, -19.75)
  line L4307 (375, 90.147) -> (309, -6)
  line L4308 (309, -6) -> (312, -6)
  line L4309 (617.8, 12) -> (747, 12)
  line L4310 (617.8, 135) -> (617.8, 132)
  line L4311 (617.8, 12) -> (617.8, 3)
  line L4312 (617.8, 79) -> (617.8, 122)
  line L4313 (627.8, 79) -> (627.8, 122)
  line L4314 (627.8, 122) -> (617.8, 122)
  line L4315 (237.7, 160.5) -> (248.2, 160.5)
  line L4316 (248.2, 160.5) -> (248.2, 150)
  line L4317 (248.2, 150) -> (237.7, 150)
  line L4318 (237.7, 150) -> (237.7, 160.5)
  line L4319 (526, 9) -> (539, 9)
  line L4320 (539, 9) -> (539, 59)
  line L4321 (539, 59) -> (526, 59)
  line L4322 (526, 59) -> (526, 9)
  arc A174 (340, 217.5) -> (340.0194, 216.3341) centre (375, 217.5) ccw
  arc A175 (340.083, 215.0916) -> (340.4891, 211.6691) centre (375, 217.5) ccw
  arc A176 (351.2448, 191.7961) -> (354.558, 189.0901) centre (375, 217.5) ccw
  arc A177 (355.5058, 188.4315) -> (357.75, 187.0461) centre (375, 217.5) ccw
  arc A178 (409.8747, 220.4591) -> (409.4268, 223.8086) centre (375, 217.5) ccw
  arc A179 (407.25, 231.0992) -> (406.4359, 232.8879) centre (375, 217.5) ccw
  arc A180 (377, 252.4428) -> (373, 252.4428) centre (375, 217.5) ccw
  arc A181 (354.558, 245.9099) -> (351.2448, 243.2039) centre (375, 217.5) ccw
  arc A182 (340, 217.5) -> (340.0194, 216.3341) centre (375, 217.5) ccw
  arc A183 (340.083, 215.0916) -> (340.4891, 211.6691) centre (375, 217.5) ccw
  arc A184 (351.2448, 191.7961) -> (354.558, 189.0901) centre (375, 217.5) ccw
  arc A185 (355.5058, 188.4315) -> (357.75, 187.0461) centre (375, 217.5) ccw
  arc A186 (354.558, -48.0901) -> (351.2448, -50.7961) centre (375, -76.5) ccw
  arc A187 (340, -76.5) -> (340.0194, -77.6659) centre (375, -76.5) ccw
  arc A188 (340.083, -78.9084) -> (340.4891, -82.3309) centre (375, -76.5) ccw
  arc A189 (351.2448, -102.2039) -> (354.558, -104.9099) centre (375, -76.5) ccw
  arc A190 (355.5058, -105.5685) -> (357.75, -106.9539) centre (375, -76.5) ccw
  arc A191 (383.427, -42.5296) -> (383.1782, -42.4689) centre (375, -76.5) ccw
  arc A192 (351.2448, -102.2039) -> (354.558, -104.9099) centre (375, -76.5) ccw
  arc A193 (355.5058, -105.5685) -> (357.75, -106.9539) centre (375, -76.5) ccw
  arc A194 (340, -76.5) -> (340.0194, -77.6659) centre (375, -76.5) ccw
  arc A195 (340.083, -78.9084) -> (340.4891, -82.3309) centre (375, -76.5) ccw
  line L4323 (383.1782, 251.5311) -> (381.25, 250.4178)
  arc A196 (383.427, 251.4704) -> (383.1782, 251.5311) centre (375, 217.5) ccw
  line L4324 (385.25, 250.4178) -> (383.427, 251.4704)
  line L4325 (385.25, 248.1084) -> (385.25, 250.4178)
  line L4326 (385.25, 250.4178) -> (383.427, 251.4704)
  line L4327 (381.25, 250.4178) -> (381.25, 248.1084)
  line L4328 (385.25, 248.1084) -> (385.25, 250.4178)
  line L4329 (383.25, 246.9537) -> (385.25, 248.1084)
  arc A197 (383.427, 251.4704) -> (383.1782, 251.5311) centre (375, 217.5) ccw
  line L4330 (381.25, 248.1084) -> (383.25, 246.9537)
  line L4331 (383.1782, 251.5311) -> (381.25, 250.4178)
  line L4332 (381.25, 248.1084) -> (383.25, 246.9537)
  line L4333 (383.25, 246.9537) -> (385.25, 248.1084)
  line L4334 (381.25, 250.4178) -> (381.25, 248.1084)
  line L4335 (617.8, 79) -> (627.8, 79)
  point P0 (375, 217.5)
  point P1 (375, 217.5)
  point P2 (375, 217.5)
  point P3 (375, 217.5)
  point P4 (375, -76.5)
  point P5 (375, -76.5)
  point P6 (375, -76.5)
  point P7 (375, -76.5)
  point P8 (751, 129.75)
  point P9 (582.2, -37.75)
  point P10 (582.2, -15.25)
  point P11 (582.2, -60.25)
  dimension "d42" = 5.5
  dimension "d43" = 0
  dimension "d46" = 5.5
  dimension "d47" = 0
  dimension "d52" = 5.5
  dimension "d53" = 0
  dimension "d56" = 5.5
  dimension "d57" = 0
  dimension "d60" = 3
  dimension "d61" = 3
  dimension "d62" = 3
  dimension "d63" = 3
  dimension "d67" = 60
  dimension "d68" = 60
  dimension "d69" = 4
  dimension "d70" = 4
  dimension "d71" = 4
  dimension "d72" = 4
  dimension "d73" = 60
  dimension "d74" = 60
  dimension "d75" = 4
  dimension "d76" = 4
  dimension "d77" = 4
  dimension "d78" = 4
  dimension "d86" = 89
  dimension "d87" = 42
  dimension "d96" = 10
  dimension "d97" = 25.5
  dimension "d98" = 10
  dimension "d99" = 25.5
  dimension "d100" = 35
  dimension "d114" = 98
  dimension "d115" = 60
  dimension "d116" = 24
  dimension "d117" = 42
  dimension "d118" = 24
  dimension "d119" = 42
  dimension "d120" = 35.5
  dimension "d121" = 38
  dimension "d122" = 10
  dimension "d123" = 25.5
  dimension "d124" = 10
  dimension "d125" = 25.5
  dimension "d126" = 34
  dimension "d127" = 128.2
  dimension "d128" = 2.5
  dimension "d129" = 112
  dimension "d131" = 2.5
  dimension "d134" = 2.5
  dimension "d137" = 2.5
  dimension "d140" = 2.5
  dimension "d149" = 2.5
  dimension "d152" = 2.5
  dimension "d153" = 2.5
  dimension "d154" = 2.5
  dimension "d161" = 115
  dimension "d168" = 3
  dimension "d169" = 3
  dimension "d170" = 3
  dimension "d171" = 3
  dimension "d212" = 22.5
  dimension "d221" = 10.5
  dimension "d222" = 10.5
  dimension "d226" = 13
  dimension "d227" = 50
  dimension "d238" = 10
  dimension "d241" = 120
  constraint coincident P3 P2
  constraint concentric A25 A174
  constraint concentric A24 A174
  constraint concentric A36 A174
  constraint coincident L1275.start A174
  constraint concentric A57 A174
  constraint coincident A45.start A174
  constraint concentric A46 A174
  constraint coincident L1465.end A174
  constraint concentric A55 A174
  constraint concentric A48 A174
  constraint coincident L1249.end A174
  constraint concentric A31 A174
  constraint concentric A29 A174
  constraint concentric A33 A174
  constraint concentric A28 A174
  constraint concentric A41 A174
  constraint concentric A67 A174
  constraint concentric A68 A174
  constraint concentric A0 A174
  constraint concentric A2 A174
  constraint concentric A34 A174
  constraint coincident L1725.end A174
  constraint concentric A64 A174
  constraint coincident A59.start A174
  constraint concentric A60 A174
  constraint concentric A8 A174
  constraint concentric A51 A174
  constraint concentric A40 A174
  constraint coincident L1408.end A174
  constraint coincident L1409.start A174
  constraint concentric A174 A176
  constraint concentric A50 A174
  constraint coincident L566.end A174
  constraint concentric A9 A174
  constraint concentric A5 A174
  constraint concentric A16 A174
  constraint coincident L615.start A174
  constraint coincident L1355.end A174
  constraint concentric A43 A174
  constraint concentric A4 A182
  constraint concentric A23 A182
  constraint concentric A22 A182
  constraint concentric A61 A182
  constraint coincident L1275.start A182
  constraint concentric A56 A182
  constraint coincident A45.start A182
  constraint concentric A45 A182
  constraint coincident L1465.end A182
  constraint concentric A52 A182
  constraint coincident L1249.end A182
  constraint concentric A30 A182
  constraint concentric A32 A182
  constraint concentric A58 A182
  constraint concentric A42 A182
  constraint concentric A66 A182
  constraint concentric A69 A182
  constraint concentric A1 A182
  constraint concentric A3 A182
  constraint concentric A35 A182
  constraint coincident L1725.end A182
  constraint concentric A65 A182
  constraint coincident A59.start A182
  constraint concentric A59 A182
  constraint concentric A7 A182
  constraint concentric A47 A182
  constraint concentric A13 A182
  constraint coincident L1408.end A182
  constraint coincident L1409.start A182
  constraint concentric A182 A184
  constraint concentric A54 A182
  constraint coincident L566.end A182
  constraint concentric A11 A182
  constraint concentric A6 A182
  constraint concentric A39 A182
  constraint coincident L615.start A182
  constraint coincident L1355.end A182
  constraint coincident L1423.start A182
  constraint concentric A44 A182
  constraint concentric A4 A12
  constraint concentric A4 A38
  constraint concentric A4 A14
  constraint concentric A4 A18
  constraint concentric A4 A17
  constraint coincident L776.start A4
  constraint coincident L695.end A4
  constraint concentric A4 A49
  constraint concentric A4 A21
  constraint concentric A4 A63
  constraint coincident L2029.start A4
  constraint coincident P7 P6
  constraint concentric A139 A187
  constraint concentric A97 A187
  constraint coincident A95.end A187
  constraint coincident A95.start A187
  constraint concentric A95 A187
  constraint concentric A96 A187
  constraint concentric A108 A187
  constraint coincident L3209.start A187
  constraint concentric A130 A187
  constraint coincident A117.start A187
  constraint concentric A118 A187
  constraint coincident L3399.end A187
  constraint concentric A127 A187
  constraint concentric A120 A187
  constraint coincident A100.start A187
  constraint concentric A103 A187
  constraint concentric A101 A187
  constraint concentric A105 A187
  constraint concentric A99 A187
  constraint concentric A113 A187
  constraint concentric A141 A187
  constraint concentric A142 A187
  constraint concentric A70 A187
  constraint concentric A72 A187
  constraint concentric A106 A187
  constraint coincident L3659.end A187
  constraint concentric A137 A187
  constraint coincident A132.start A187
  constraint concentric A133 A187
  constraint concentric A78 A187
  constraint concentric A123 A187
  constraint concentric A112 A187
  constraint coincident L3342.end A187
  constraint coincident L3343.start A187
  constraint concentric A187 A192
  constraint concentric A122 A187
  constraint coincident L2490.end A187
  constraint concentric A79 A187
  constraint concentric A75 A187
  constraint concentric A86 A187
  constraint coincident L2539.start A187
  constraint coincident L3289.end A187
  constraint concentric A115 A187
  constraint concentric A80 A139
  constraint concentric A109 A139
  constraint concentric A85 A139
  constraint concentric A91 A139
  constraint concentric A98 A139
  constraint coincident A89.end A139
  constraint coincident L2619.end A139
  constraint concentric A125 A139
  constraint concentric A90 A139
  constraint concentric A135 A139
  constraint concentric A74 A194
  constraint concentric A94 A194
  constraint coincident A95.end A194
  constraint coincident A95.start A194
  constraint concentric A93 A194
  constraint concentric A134 A194
  constraint coincident L3209.start A194
  constraint concentric A129 A194
  constraint coincident A117.start A194
  constraint concentric A117 A194
  constraint coincident L3399.end A194
  constraint concentric A128 A194
  constraint concentric A124 A194
  constraint coincident A100.start A194
  constraint concentric A100 A194
  constraint concentric A102 A194
  constraint concentric A104 A194
  constraint concentric A131 A194
  constraint concentric A114 A194
  constraint concentric A140 A194
  constraint concentric A143 A194
  constraint concentric A71 A194
  constraint concentric A73 A194
  constraint concentric A107 A194
  constraint coincident L3659.end A194
  constraint concentric A138 A194
  constraint coincident A132.start A194
  constraint concentric A132 A194
  constraint concentric A77 A194
  constraint concentric A119 A194
  constraint concentric A83 A194
  constraint coincident L3342.end A194
  constraint coincident L3343.start A194
  constraint concentric A189 A194
  constraint concentric A126 A194
  constraint coincident L2490.end A194
  constraint concentric A81 A194
  constraint concentric A76 A194
  constraint concentric A111 A194
  constraint coincident L2539.start A194
  constraint coincident L3289.end A194
  constraint coincident L3357.start A194
  constraint concentric A116 A194
  constraint concentric A74 A82
  constraint concentric A74 A110
  constraint concentric A74 A84
  constraint concentric A74 A88
  constraint concentric A74 A87
  constraint coincident A89.end A74
  constraint concentric A74 A89
  constraint coincident L2619.end A74
  constraint concentric A74 A121
  constraint concentric A74 A92
  constraint concentric A74 A136
  constraint coincident L3963.start A74
  constraint horizontal L4220
  constraint vertical L4221
  constraint horizontal L4222
  constraint vertical L4223
  constraint horizontal L4224
  constraint vertical L4225
  constraint horizontal L4226
  constraint vertical L4227
  constraint horizontal L4228
  constraint vertical L4229
  constraint horizontal L4230
  constraint vertical L4231
  constraint horizontal L4232
  constraint horizontal L4271
  constraint vertical L4258
  constraint horizontal L4260
  constraint vertical L4252
  constraint horizontal L4266
  constraint vertical L4264
  constraint horizontal L4254
  constraint vertical L4275
  constraint horizontal L4273
  constraint vertical L4280
  constraint horizontal L4255
  constraint vertical L4253
  constraint midpoint L4272.start L4252
  constraint midpoint L4272.end L4258
  constraint midpoint L4270.start L4260
  constraint midpoint L4270.end L4271
  constraint midpoint L4263.start L4275
  constraint midpoint L4263.end L4264
  constraint midpoint L4269.start L4266
  constraint midpoint L4269.end L4254
  constraint midpoint L4278.start L4253
  constraint midpoint L4278.end L4280
  constraint midpoint L4268.start L4273
  constraint midpoint L4268.end L4255
  constraint horizontal L4257
  constraint vertical L4276
  constraint horizontal L4248
  constraint vertical L4265
  constraint midpoint L4282.start L4265
  constraint midpoint L4282.end L4276
  constraint midpoint L4262.start L4257
  constraint midpoint L4262.end L4248
  constraint horizontal L4249
  constraint vertical L4279
  constraint horizontal L4267
  constraint vertical L4281
  constraint midpoint L4269.end L4249
  constraint horizontal L4259
  constraint vertical L4250
  constraint horizontal L4247
  constraint vertical L4277
  constraint midpoint L4268.end L4247
  constraint midpoint A161.centre L4262
  constraint horizontal L4261
  constraint vertical L4256
  constraint horizontal L4251
  constraint vertical L4274
  constraint vertical L4235
  constraint perpendicular L4283 L4289
  constraint vertical L4283
  constraint perpendicular L209 L4301
  constraint perpendicular L106 L4302
  constraint perpendicular L4284 L4303
  constraint perpendicular L4303 L4304
  constraint perpendicular L4304 L4305
  constraint perpendicular L132 L4310
  constraint parallel L4310 L4311
  constraint horizontal L4314
  constraint horizontal L4315
  constraint vertical L4316
  constraint horizontal L4317
  constraint vertical L4318
  constraint horizontal L4319
  constraint vertical L4320
  constraint horizontal L4321
  constraint vertical L4322
  constraint concentric A174 A175
  constraint concentric A176 A177
  constraint concentric A182 A183
  constraint concentric A184 A185
  constraint concentric A187 A188
  constraint concentric A189 A190
  constraint concentric A192 A193
  constraint concentric A194 A195
  constraint perpendicular L4313 L4335
  measures "d60" diameter of A150
  measures "d61" diameter of A149
  measures "d62" diameter of A147
  measures "d63" diameter of A148
  measures "d67" distance of A152.centre A153.centre
  measures "d68" distance of A153.centre A154.centre
  measures "d69" diameter of A152
  measures "d70" diameter of A153
  measures "d71" diameter of A154
  measures "d72" diameter of A155